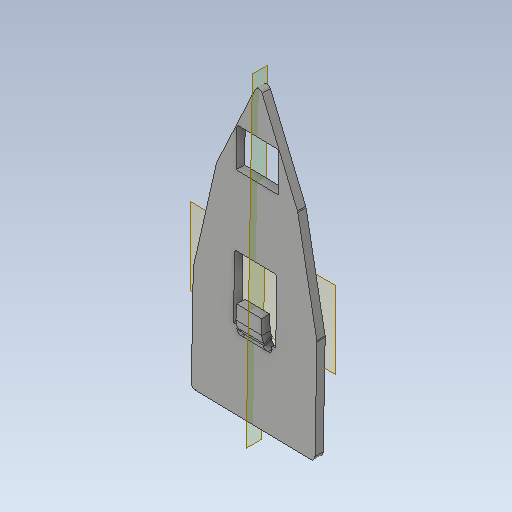
# Autodesk Inventor part: top vange-endeplade
Saved by Autodesk Inventor 2020.1 (Build 241239000, 239)
## iProperties
Created: 2019-09-25
Part Number: top vange-endeplade
Material: S235JR
Document SubType Name: Sheet Metal
Designer: gust3763
Density: 7.85 g/cm^3
Sheet Metal Rule: Default_mm
Appearance: Light Gray
Mass: 1385.49 g
Surface Area: 533.226 cm^2
Volume: 176.496 cm^3
Flat Pattern Width: 28.5453 cm
Flat Pattern Length: 12 cm
Flat Pattern Area: 342.544 cm^2
Sheet Metal Width: 285,453 mm
Sheet Metal Length: 120,000 mm
Sheet Metal Area: 34254,356 mm^2
Author: gust3763
Autodesk Inventor part; units mm, degrees
ref_plane "YZ Plane" through (0, 0, 0) normal (1, 0, 0) x (0, 1, 0)
ref_plane "XZ Plane" through (0, 0, 0) normal (0, 1, 0) x (-1, 0, 0)
ref_plane "XY Plane" through (0, 0, 0) normal (0, 0, 1) x (1, 0, 0)
ref_plane "Work Plane1" through (0, 7.8369, -252.3493) normal (0, 0, 1) x (1, 0, 0)
sketch "Sketch1" plane through (0, 7.8369, -252.3493) normal (0, 0, 1) x (1, 0, 0)
  line L0 (80.2691, 112.9923) -> (81.4188, 172.9812)
  line L1 (79.4575, 175.0192) -> (42.4643, 175.7282)
  line L2 (40.4263, 173.7668) -> (39.2766, 113.7779)
  line L3 (46.7753, 113.6342) -> (48.2349, 137.6106)
  line L4 (48.2349, 137.6106) -> (72.2305, 137.1507)
  line L5 (72.2305, 137.1507) -> (72.7705, 113.136)
  line L6 (39.2766, 113.7779) -> (46.7753, 113.6342)
  line L7 (72.7705, 113.136) -> (80.2691, 112.9923)
  arc A0 (81.4188, 172.9812) -> (79.4575, 175.0192) centre (79.4191, 173.0196) ccw
  arc A1 (42.4643, 175.7282) -> (40.4263, 173.7668) centre (42.4259, 173.7285) ccw
  line L8 (82.5101, 242.9732) -> (42.0175, 243.7492)
  line L9 (42.0175, 243.7492) -> (42.7073, 279.7426)
  line L10 (44.7453, 281.7039) -> (81.2386, 281.0045)
  line L11 (83.1999, 278.9666) -> (82.5101, 242.9732)
  arc A2 (83.1999, 278.9666) -> (81.2386, 281.0045) centre (81.2003, 279.0049) ccw
  arc A3 (44.7453, 281.7039) -> (42.7073, 279.7426) centre (44.707, 279.7043) ccw
  ellipse E0 centre (114.6452, 40.9624) end of major axis (114.4887, 32.7929) minor radius 6.75 (114.4887, 32.7929) -> (121.394, 40.833) ccw
  line L12 (123.2562, 138.0026) -> (121.394, 40.833)
  ellipse E1 centre (116.5075, 138.132) end of major axis (116.664, 146.3014) minor radius 6.75 (123.2562, 138.0026) -> (123.0912, 139.9961) ccw
  line L13 (104.6213, 238.4876) -> (123.0912, 139.9961)
  ellipse E2 centre (98.0376, 236.6234) end of major axis (98.1941, 244.7929) minor radius 6.75 (104.6213, 238.4876) -> (104.0597, 240.3689) ccw
  line L14 (69.7234, 322.109) -> (104.0597, 240.3689)
  ellipse E3 centre (63.7012, 318.3636) end of major axis (63.8578, 326.533) minor radius 6.75 (69.7234, 322.109) -> (57.827, 322.337) ccw
  line L15 (20.384, 241.9725) -> (57.827, 322.337)
  ellipse E4 centre (26.2582, 237.9991) end of major axis (26.4148, 246.1685) minor radius 6.75 (20.384, 241.9725) -> (19.7508, 240.1141) ccw
  line L16 (-2.4793, 142.4027) -> (19.7508, 240.1141)
  ellipse E5 centre (4.0281, 140.2876) end of major axis (4.1847, 148.457) minor radius 6.75 (-2.4793, 142.4027) -> (-2.7206, 140.4169) ccw
  line L17 (-4.5829, 43.2473) -> (-2.7206, 140.4169)
  ellipse E6 centre (2.1659, 43.118) end of major axis (2.0093, 34.9486) minor radius 6.75 (-4.5829, 43.2473) -> (2.0093, 34.9486) ccw
  line L18 (2.0093, 34.9486) -> (56.7493, 33.8995)
  line L19 (56.8189, 37.5303) -> (56.7493, 33.8995)
  line L20 (2.0789, 38.5794) -> (56.8189, 37.5303)
  ellipse E7 centre (2.1659, 43.118) end of major axis (2.0789, 38.5794) minor radius 3.75 (-1.5834, 43.1899) -> (2.0789, 38.5794) ccw
  line L21 (0.2788, 140.3594) -> (-1.5834, 43.1899)
  ellipse E8 centre (4.0281, 140.2876) end of major axis (4.1151, 144.8262) minor radius 3.75 (0.4129, 141.4626) -> (0.2788, 140.3594) ccw
  line L22 (22.643, 239.1741) -> (0.4129, 141.4626)
  ellipse E9 centre (26.2582, 237.9991) end of major axis (26.3452, 242.5376) minor radius 3.75 (22.9947, 240.2065) -> (22.643, 239.1741) ccw
  line L23 (60.4378, 320.571) -> (22.9947, 240.2065)
  ellipse E10 centre (63.7012, 318.3636) end of major axis (63.7882, 322.9022) minor radius 3.75 (67.0469, 320.4444) -> (60.4378, 320.571) ccw
  line L24 (101.3832, 238.7042) -> (67.0469, 320.4444)
  ellipse E11 centre (98.0376, 236.6234) end of major axis (98.1245, 241.162) minor radius 3.75 (101.6952, 237.6591) -> (101.3832, 238.7042) ccw
  line L25 (120.1651, 139.1676) -> (101.6952, 237.6591)
  ellipse E12 centre (116.5075, 138.132) end of major axis (116.5945, 142.6705) minor radius 3.75 (120.2568, 138.0601) -> (120.1651, 139.1676) ccw
  line L26 (118.3946, 40.8905) -> (120.2568, 138.0601)
  ellipse E13 centre (114.6452, 40.9624) end of major axis (114.5583, 36.4238) minor radius 3.75 (114.5583, 36.4238) -> (118.3946, 40.8905) ccw
  line L27 (59.8183, 37.4729) -> (114.5583, 36.4238)
  line L28 (59.7487, 33.842) -> (59.8183, 37.4729)
  line L29 (59.7487, 33.842) -> (114.4887, 32.7929)
  line L30 (59.8183, 37.4729) -> (56.8189, 37.5303)
  line L31 (54.6555, -153.6335) -> (79.6842, 1152.3434) construction
  point P0 (81.4571, 174.9809)
  point P1 (40.4646, 175.7665)
  point P2 (83.2382, 280.9662)
  dimension "d9" = 41
  dimension "d10" = 24
  dimension "d11" = 38
  dimension "d12" = 24
  dimension "d13" = 26
  dimension "d14" = 2
  dimension "d22" = 130
  dimension "d23" = 40.5
  dimension "d24" = 38
  dimension "d25" = 2
  dimension "d28" = 3
  measures "d9" distance of point (81.457, 174.981) point (40.465, 175.766)
  measures "d10" distance of L4.start L4.end
  measures "d11" distance between parallel lines of L1 L4
  measures "d12" distance between parallel lines of L7 L4
  measures "d13" distance of L5.end L3.start
  measures "d14" radius of A0
  measures "d22" distance between parallel lines of L8 L6
  measures "d23" distance between parallel lines of L9 L11
  measures "d24" distance of point (83.238, 280.966) L8.start
  measures "d25" radius of A2
  measures "d28" distance from line of A2.centre L24
extrude "Plate1" add sketch "Sketch1" along normal blind 8 contours L30 L20 E7 L21 E8 L22 E9 L23 E10 L24 E11 L25 E12 L26 E13 L27
hole "Hole1" at (72.838, 117.9711, -244.3493) direction (0, 0, -1) diameter 8 depth 8 tip angle 118
hole "Hole2" at (46.5928, 118.474, -244.3493) direction (0, 0, -1) diameter 8 depth 8 tip angle 118
fillet "Fillet1" radius 1 4 edges at (75.5407, 120.9198, -248.3493) (72.7481, 121.97, -248.3493) (44.005, 121.5242, -248.3493) (46.8359, 122.4666, -248.3493)
sketch "Sketch2" plane through (0, 7.8369, -244.3493) normal (0, 0, 1) x (1, 0, 0)
  arc A0 (71.9501, 114.0343) -> (76.534, 111.6636) centre (72.838, 110.1341) ccw projected
  arc A1 (42.9581, 112.3071) -> (47.6295, 114.5004) centre (46.5928, 110.6371) ccw projected
  line L0 (72.2305, 137.1507) -> (48.2349, 137.6106) projected
  line L1 (72.7613, 106.1349) -> (46.5162, 106.6378)
  point P0 (0, -7.8369)
  constraints: 2 end point, 2 point on circle, 1 parallel, 1 tangent
fold "Fold1" angle 30 bend radius 8 thickness 8 k factor 0.44 line from (72.7613, 113.9718, -244.3493) to (46.5162, 114.4748, -244.3493) line at bend start moving side (0.0191612, 0.9998164, 0) folds toward (0, 0, 1)
sketch "Sketch3" plane through (72.2042, 143.611, -237.7216) normal (0.0095806, 0.4999082, -0.8660254) x (-0.9998164, 0.0191612, 0)
  line L0 (0, 0) -> (-0.9211, -22.1053) projected
  line L1 (24.9211, -22.1053) -> (24, 0) projected
  line L2 (24, 0) -> (0, 0) projected
  line L3 (-0.8333, -20) -> (24.8333, -20)
  point P0 (69.4391, -6.6852)
  dimension "d54" = 20
  constraints: 2 end point, 2 point on line, 1 parallel
  measures "d54" distance between parallel lines of L2 L3
fold "Fold2" angle 30 bend radius 8 thickness 8 k factor 0.44 line from (72.7055, 126.2777, -247.7216) to (47.0435, 126.7695, -247.7216) line at bend start moving side (0.0165941, 0.8658664, 0.5) folds toward (0.0095806, 0.4999082, -0.8660254)
ref_plane "modtplan" through (60.2678, 147.0467, -252.3493) normal (-0.9998164, 0.0191612, 0) x (0, 0, 1)
equation "\"d24\" = d11"
equation "\"d0\" = Thickness"
equation "\"BendRadius\" = Thickness"
equation "\"BendReliefWidth\" = Thickness"
equation "\"BendReliefDepth\" = 0.5 * Thickness"
equation "\"CornerReliefSize\" = 4 * Thickness"
equation "\"MinimumRemnant\" = 2 * Thickness"
equation "\"TransitionRadius\" = BendRadius"
equation "\"JacobiRadiusSize\" = BendRadius"
equation "\"GapSize\" = Thickness"
equation "\"Thickness\" = 8"
body "Solid1"
